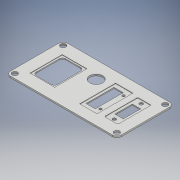
# Autodesk Inventor part: Paneeltje
Saved by Autodesk Inventor 2018 (Build 220112000, 112)
## iProperties
Created: 2018-02-27
Part Number: Paneeltje
Material: Generic
Document SubType Name: Modeling
Designer: Dieter Vansteenwegen
Density: 1 g/cm^3
Appearance: Default
Author: Dieter Vansteenwegen
Autodesk Inventor part; units mm, degrees
ref_plane "YZ Plane" through (0, 0, 0) normal (1, 0, 0) x (0, 1, 0)
ref_plane "XZ Plane" through (0, 0, 0) normal (0, 1, 0) x (-1, 0, 0)
ref_plane "XY Plane" through (0, 0, 0) normal (0, 0, 1) x (1, 0, 0)
sketch "Sketch1" plane through (0, 0, 0) normal (0, 0, 1) x (1, 0, 0)
  line L0 (-47.5, 26.5) -> (47.5, 26.5)
  line L1 (51.5, 22.5) -> (51.5, -22.5)
  line L2 (47.5, -26.5) -> (-47.5, -26.5)
  line L3 (-51.5, -22.5) -> (-51.5, 22.5)
  arc A0 (-51.5, -22.5) -> (-47.5, -26.5) centre (-47.5, -22.5) ccw
  arc A1 (47.5, -26.5) -> (51.5, -22.5) centre (47.5, -22.5) ccw
  arc A2 (51.5, 22.5) -> (47.5, 26.5) centre (47.5, 22.5) ccw
  arc A3 (-47.5, 26.5) -> (-51.5, 22.5) centre (-47.5, 22.5) ccw
  line L4 (-47.51, 22.5) -> (47.51, 22.5) construction
  line L5 (47.51, 22.5) -> (47.51, -22.5) construction
  line L6 (47.51, -22.5) -> (-47.51, -22.5) construction
  line L7 (-47.51, -22.5) -> (-47.51, 22.5) construction
  circle A4 centre (-47.51, 22.5) radius 2.5
  circle A5 centre (47.51, 22.5) radius 2.5
  circle A6 centre (-47.51, -22.5) radius 2.5
  circle A7 centre (47.51, -22.5) radius 2.5
  point P0 (0, 0)
  point P1 (-51.5, 26.5)
  point P2 (51.5, -26.5)
  point P3 (51.5, 26.5)
  point P4 (0, 26.5)
  point P5 (51.5, 0)
  point P6 (47.51, 0)
  point P7 (0, 22.5)
  dimension "d0" = 103
  dimension "d1" = 53
  dimension "d3" = 4
  dimension "d4" = 95.02
  dimension "d5" = 45
  dimension "d6" = 5
  dimension "d7" = 5
  dimension "d8" = 5
  dimension "d9" = 5
  constraints: 16 end point, 8 centre point, 8 point on circle, 8 tangent, 6 point on line, 4 coincident, 4 midpoint, 4 parallel, 3 equal radius, 2 horizontal, 2 horizontal alignment, 2 perpendicular, 2 vertical alignment
  measures "d0" distance of point (-51.5, 26.5) point (51.5, 26.5)
  measures "d1" distance of point (51.5, 26.5) point (51.5, -26.5)
  measures "d3" radius of A0
  measures "d4" distance of L4.start L4.end
  measures "d5" distance of L4.end L5.end
  measures "d6" diameter of A4
  measures "d7" diameter of A5
  measures "d8" diameter of A6
  measures "d9" diameter of A7
extrude "Extrusion1" add sketch "Sketch1" along normal mid plane 1.5
sketch "Sketch2" plane through (0, 0, 0.75) normal (0, 0, 1) x (1, 0, 0)
  line L0 (47.5, 26.5) -> (-47.5, 26.5) projected
  point P0 (0, 0)
  point P1 (-5, 10.8)
  dimension "d51" = 5
  dimension "d52" = 15.7
  measures "d51" horizontal distance of point (0, 0) point (-5, 10.8)
  measures "d52" distance from line of point (-5, 10.8) L0
hole "Neon" at (-5, 10.8, 0.75) direction (0, 0, -1) diameter 12 end through all
sketch "Sketch3" plane through (0, 0, 0.75) normal (0, 0, 1) x (1, 0, 0)
  line L0 (-36.3319, 13.6885) -> (-22.3319, 13.6885)
  line L1 (-19.3319, 10.6885) -> (-19.3319, -10.8115)
  line L2 (-22.3319, -13.8115) -> (-36.3319, -13.8115)
  line L3 (-39.3319, -10.8115) -> (-39.3319, 10.6885)
  arc A0 (-36.3319, 13.6885) -> (-39.3319, 10.6885) centre (-36.3319, 10.6885) ccw
  arc A1 (-19.3319, 10.6885) -> (-22.3319, 13.6885) centre (-22.3319, 10.6885) ccw
  arc A2 (-22.3319, -13.8115) -> (-19.3319, -10.8115) centre (-22.3319, -10.8115) ccw
  arc A3 (-39.3319, -10.8115) -> (-36.3319, -13.8115) centre (-36.3319, -10.8115) ccw
  line L4 (-40.8319, 14.9385) -> (-17.8319, 14.9385)
  line L5 (-17.8319, 14.9385) -> (-17.8319, -15.0615)
  line L6 (-17.8319, -15.0615) -> (-40.8319, -15.0615)
  line L7 (-40.8319, -15.0615) -> (-40.8319, 14.9385)
  point P0 (0, 0)
  point P1 (-39.3319, 13.6885)
  point P2 (-19.3319, -13.8115)
  point P3 (-19.3319, 13.6885)
  point P4 (-17.8319, -0.0615)
  point P5 (-19.3319, -0.0615)
  point P6 (-29.3319, 14.9385)
  point P7 (-29.3319, 13.6885)
  dimension "d20" = 20
  dimension "d21" = 27.5
  dimension "d22" = 3
  dimension "d37" = 30
  dimension "d38" = 23
  constraints: 16 end point, 8 point on circle, 8 tangent, 6 point on line, 4 centre point, 4 midpoint, 4 parallel, 3 equal radius, 2 horizontal, 2 perpendicular, 1 horizontal alignment, 1 vertical alignment
  measures "d20" distance of point (-39.332, 13.689) point (-19.332, 13.689)
  measures "d21" distance of point (-19.332, 13.689) point (-19.332, -13.811)
  measures "d22" radius of A0
  measures "d37" distance of L4.end L5.end
  measures "d38" distance of L4.start L4.end
extrude "IEC" cut sketch "Sketch3" against normal through all contours L0 A1 L1 A2 L2 A3 L3 A0
sketch "Sketch4" plane through (0, 0, 0.75) normal (0, 0, 1) x (1, 0, 0)
  line L0 (39.1106, 8.15) -> (31.2106, 8.15)
  line L1 (31.2106, 8.15) -> (31.2106, -8.15)
  line L2 (31.2106, -8.15) -> (39.1106, -8.15)
  line L3 (39.1106, -8.15) -> (39.1106, 8.15)
  circle A0 centre (35.1606, 12.5) radius 1.55
  circle A1 centre (35.1606, -12.5) radius 1.55
  line L4 (35.1606, 12.5) -> (35.1606, -12.5) construction
  line L5 (29.9106, 15.5) -> (40.4106, 15.5)
  line L6 (41.4106, 14.5) -> (41.4106, -14.5)
  line L7 (40.4106, -15.5) -> (29.9106, -15.5)
  line L8 (28.9106, -14.5) -> (28.9106, 14.5)
  arc A2 (41.4106, 14.5) -> (40.4106, 15.5) centre (40.4106, 14.5) ccw
  arc A3 (29.9106, 15.5) -> (28.9106, 14.5) centre (29.9106, 14.5) ccw
  arc A4 (28.9106, -14.5) -> (29.9106, -15.5) centre (29.9106, -14.5) ccw
  arc A5 (40.4106, -15.5) -> (41.4106, -14.5) centre (40.4106, -14.5) ccw
  point P0 (0, 0)
  point P1 (35.1606, 8.15)
  point P2 (35.1606, -8.15)
  point P3 (35.1606, 0)
  point P4 (39.1106, 0)
  point P5 (41.4106, 0)
  point P6 (35.1606, 15.5)
  dimension "d25" = 7.9
  dimension "d26" = 16.3
  dimension "d27" = 3.1
  dimension "d28" = 3.1
  dimension "d29" = 25
  dimension "d30" = 1
  dimension "d31" = 31
  dimension "d32" = 12.5
  constraints: 18 end point, 8 point on circle, 8 tangent, 6 centre point, 6 midpoint, 4 parallel, 3 equal radius, 3 horizontal alignment, 3 vertical alignment, 2 horizontal, 2 perpendicular, 1 vertical
  measures "d25" distance of L0.start L0.end
  measures "d26" distance of L2.end L0.start
  measures "d27" diameter of A0
  measures "d28" diameter of A1
  measures "d29" distance of L4.end L4.start
  measures "d30" radius of A2
  measures "d31" distance between parallel lines of L7 L5
  measures "d32" distance between parallel lines of L6 L8
extrude "SUB-D" cut sketch "Sketch4" against normal through all contours L3 L2 L1 L0 | A0 | A1
extrude "Extrusion4" cut sketch "Sketch4" against normal blind 0.5
extrude "Extrusion5" cut sketch "Sketch3" against normal blind 0.5
sketch "Sketch5" plane through (0, 0, 0.75) normal (0, 0, 1) x (1, 0, 0)
  line L0 (7.0815, 16.72) -> (23.2815, 16.72)
  line L1 (23.2815, 16.72) -> (23.2815, -16.72)
  line L2 (23.2815, -16.72) -> (7.0815, -16.72)
  line L3 (7.0815, -16.72) -> (7.0815, 16.72)
  line L4 (9.2315, 13.05) -> (17.9315, 13.05)
  line L5 (17.9315, 13.05) -> (17.9315, -13.05)
  line L6 (17.9315, -13.05) -> (9.2315, -13.05)
  line L7 (9.2315, -13.05) -> (9.2315, 13.05)
  line L8 (20.4815, 10.715) -> (20.4815, -10.715) construction
  circle A0 centre (20.4815, 10.715) radius 1.15
  circle A1 centre (20.4815, -10.715) radius 1.15
  point P0 (0, 0)
  point P1 (17.9315, 0)
  point P2 (23.2815, 0)
  point P3 (20.4815, 0)
  point P4 (7.0815, 0)
  dimension "d41" = 16.2
  dimension "d42" = 33.44
  dimension "d43" = 8.7
  dimension "d44" = 14.05
  dimension "d45" = 2.8
  dimension "d46" = 21.43
  dimension "d47" = 26.1
  dimension "d48" = 2.3
  dimension "d49" = 2.3
  constraints: 18 end point, 4 midpoint, 4 parallel, 3 horizontal alignment, 2 centre point, 2 coincident, 2 horizontal, 2 perpendicular, 1 vertical
  measures "d41" distance of L0.start L0.end
  measures "d42" distance of L0.end L1.end
  measures "d43" distance of L4.start L4.end
  measures "d44" distance between parallel lines of L1 L7
  measures "d45" distance between parallel lines of L1 L8
  measures "d46" distance of L8.start L8.end
  measures "d47" distance of L6.end L4.start
  measures "d48" diameter of A0
  measures "d49" diameter of A1
extrude "Extrusion6" cut sketch "Sketch5" against normal through all contours L4 L5 L6 L7 | A0 | A1
extrude "Extrusion7" cut sketch "Sketch5" against normal blind 0.5
body "Solid1"
